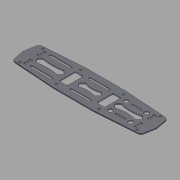
# Autodesk Inventor part: Top Plate
Saved by Autodesk Inventor 2011 SP2 (Build 150309200, 309)
## iProperties
Created: 2015-02-19
Part Number: Top Plate
Document SubType Name: Modeling
Designer: Greg Pavlik
Density: 1 g/cm^3
Author: Greg Pavlik
Autodesk Inventor part; units mm, degrees
ref_plane "YZ Plane" through (0, 0, 0) normal (1, 0, 0) x (0, 1, 0)
ref_plane "XZ Plane" through (0, 0, 0) normal (0, 1, 0) x (-1, 0, 0)
ref_plane "XY Plane" through (0, 0, 0) normal (0, 0, 1) x (1, 0, 0)
sketch "Sketch1" plane through (0, 0, 0) normal (0, 0, 1) x (1, 0, 0)
  line L0 (-92, 0) -> (92, 0) construction
  line L1 (0, 23) -> (0, -23) construction
  line L2 (26.8254, 23) -> (-26.8254, 23)
  line L3 (-27.1742, 22.9878) -> (-84.8084, 18.9576)
  line L4 (-89.3836, 14.8381) -> (-91.8469, 0.8682)
  line L5 (27.1742, 22.9878) -> (84.8084, 18.9576)
  line L6 (89.3836, 14.8381) -> (91.8469, 0.8682)
  line L7 (26.8254, -23) -> (-26.8254, -23)
  line L8 (-27.1742, -22.9878) -> (-84.8084, -18.9576)
  line L9 (-89.3836, -14.8381) -> (-91.8469, -0.8682)
  line L10 (89.3836, -14.8381) -> (91.8469, -0.8682)
  line L11 (27.1742, -22.9878) -> (84.8084, -18.9576)
  arc A0 (-84.8084, 18.9576) -> (-89.3836, 14.8381) centre (-84.4596, 13.9698) ccw
  arc A1 (-26.8254, 23) -> (-27.1742, 22.9878) centre (-26.8254, 18) ccw
  arc A2 (-91.8469, 0.8682) -> (-91.8469, -0.8682) centre (-86.9229, 0) ccw
  arc A3 (-89.3836, -14.8381) -> (-84.8084, -18.9576) centre (-84.4596, -13.9698) ccw
  arc A4 (-27.1742, -22.9878) -> (-26.8254, -23) centre (-26.8254, -18) ccw
  arc A5 (26.8254, -23) -> (27.1742, -22.9878) centre (26.8254, -18) ccw
  arc A6 (84.8084, -18.9576) -> (89.3836, -14.8381) centre (84.4596, -13.9698) ccw
  arc A7 (91.8469, -0.8682) -> (91.8469, 0.8682) centre (86.9229, 0) ccw
  arc A8 (89.3836, 14.8381) -> (84.8084, 18.9576) centre (84.4596, 13.9698) ccw
  arc A9 (27.1742, 22.9878) -> (26.8254, 23) centre (26.8254, 18) ccw
  point P0 (0, 0)
  point P1 (27, 23)
  point P2 (-27, 23)
  point P3 (-88.7053, 18.6851)
  point P4 (88.7053, 18.6851)
  point P5 (27, -23)
  point P6 (-27, -23)
  point P7 (-88.7053, -18.6851)
  point P8 (88.7053, -18.6851)
  dimension "d0" = 184
  dimension "d1" = 54
  dimension "d2" = 46
  dimension "d3" = 160
  dimension "d4" = 8
  dimension "d5" = 5
  constraints: 24 end point, 20 point on circle, 20 point on line, 20 tangent, 10 centre point, 9 equal radius, 7 symmetric about line, 4 midpoint, 2 perpendicular, 1 horizontal
  measures "d0" distance of L0.end L0.start
  measures "d1" distance of point (27, -23) point (-27, -23)
  measures "d2" distance between parallel lines of L2 L7
  measures "d3" angle of L10 L6
  measures "d4" angle of L8 L3
  measures "d5" radius of A0
extrude "Extrusion1" add sketch "Sketch1" along normal mid plane 1.5
sketch "Sketch2" plane through (0, 0, 0.75) normal (0, 0, 1) x (1, 0, 0)
  arc A0 (-91.8469, 0.8682) -> (-91.8469, -0.8682) centre (-86.9229, 0) ccw construction
  line L0 (26.8254, -23) -> (-26.8254, -23) construction
  arc A1 (91.8469, -0.8682) -> (91.8469, 0.8682) centre (86.9229, 0) ccw construction
  line L1 (-26.8254, 23) -> (26.8254, 23) construction
  line L2 (-91.9229, 0) -> (91.9229, 0) construction
  line L3 (0, -23) -> (0, 23) construction
  line L4 (-13, 11.5) -> (13, 11.5)
  line L5 (13, 14.5) -> (-13, 14.5)
  arc A2 (-13, 14.5) -> (-13, 11.5) centre (-13, 13) ccw
  arc A3 (13, 11.5) -> (13, 14.5) centre (13, 13) ccw
  line L6 (-13, -11.5) -> (13, -11.5)
  line L7 (13, -14.5) -> (-13, -14.5)
  arc A4 (-13, -11.5) -> (-13, -14.5) centre (-13, -13) ccw
  arc A5 (13, -14.5) -> (13, -11.5) centre (13, -13) ccw
  line L8 (-30.5, -11.25) -> (-21.5, -11.25)
  line L9 (-20.5, -10.25) -> (-20.5, 10.25)
  line L10 (-21.5, 11.25) -> (-30.5, 11.25)
  line L11 (-31.5, 10.25) -> (-31.5, -10.25)
  arc A6 (-31.5, -10.25) -> (-30.5, -11.25) centre (-30.5, -10.25) ccw
  arc A7 (-21.5, -11.25) -> (-20.5, -10.25) centre (-21.5, -10.25) ccw
  arc A8 (-20.5, 10.25) -> (-21.5, 11.25) centre (-21.5, 10.25) ccw
  arc A9 (-30.5, 11.25) -> (-31.5, 10.25) centre (-30.5, 10.25) ccw
  line L12 (30.5, -11.25) -> (21.5, -11.25)
  line L13 (20.5, -10.25) -> (20.5, 10.25)
  line L14 (21.5, 11.25) -> (30.5, 11.25)
  line L15 (31.5, 10.25) -> (31.5, -10.25)
  arc A10 (30.5, -11.25) -> (31.5, -10.25) centre (30.5, -10.25) ccw
  arc A11 (20.5, -10.25) -> (21.5, -11.25) centre (21.5, -10.25) ccw
  arc A12 (21.5, 11.25) -> (20.5, 10.25) centre (21.5, 10.25) ccw
  arc A13 (31.5, 10.25) -> (30.5, 11.25) centre (30.5, 10.25) ccw
  line L16 (-77, 4.5) -> (-75, 4.5)
  line L17 (-75, 6.5) -> (-75, 12.5)
  line L18 (-75, 14.5) -> (-77, 14.5)
  line L19 (-77, 12.5) -> (-77, 6.5)
  arc A14 (-75, 4.5) -> (-75, 6.5) centre (-75, 5.5) ccw
  arc A15 (-75, 12.5) -> (-75, 14.5) centre (-75, 13.5) ccw
  arc A16 (-77, 14.5) -> (-77, 12.5) centre (-77, 13.5) ccw
  arc A17 (-77, 6.5) -> (-77, 4.5) centre (-77, 5.5) ccw
  line L20 (-77, -4.5) -> (-75, -4.5)
  line L21 (-75, -6.5) -> (-75, -12.5)
  line L22 (-75, -14.5) -> (-77, -14.5)
  line L23 (-77, -12.5) -> (-77, -6.5)
  arc A18 (-75, -6.5) -> (-75, -4.5) centre (-75, -5.5) ccw
  arc A19 (-75, -14.5) -> (-75, -12.5) centre (-75, -13.5) ccw
  arc A20 (-77, -12.5) -> (-77, -14.5) centre (-77, -13.5) ccw
  arc A21 (-77, -4.5) -> (-77, -6.5) centre (-77, -5.5) ccw
  line L24 (77, 4.5) -> (75, 4.5)
  line L25 (75, 6.5) -> (75, 12.5)
  line L26 (75, 14.5) -> (77, 14.5)
  line L27 (77, 12.5) -> (77, 6.5)
  arc A22 (75, 6.5) -> (75, 4.5) centre (75, 5.5) ccw
  arc A23 (75, 14.5) -> (75, 12.5) centre (75, 13.5) ccw
  arc A24 (77, 12.5) -> (77, 14.5) centre (77, 13.5) ccw
  arc A25 (77, 4.5) -> (77, 6.5) centre (77, 5.5) ccw
  arc A26 (75, -4.5) -> (75, -6.5) centre (75, -5.5) ccw
  line L28 (75, -6.5) -> (75, -12.5)
  line L29 (77, -4.5) -> (75, -4.5)
  line L30 (77, -12.5) -> (77, -6.5)
  arc A27 (77, -6.5) -> (77, -4.5) centre (77, -5.5) ccw
  line L31 (75, -14.5) -> (77, -14.5)
  arc A28 (77, -14.5) -> (77, -12.5) centre (77, -13.5) ccw
  arc A29 (75, -12.5) -> (75, -14.5) centre (75, -13.5) ccw
  line L32 (47, 10) -> (59.5, 10)
  line L33 (59.5, 12) -> (47, 12)
  arc A30 (47, 12) -> (47, 10) centre (47, 11) ccw
  arc A31 (59.5, 10) -> (59.5, 12) centre (59.5, 11) ccw
  line L34 (47, -10) -> (59.5, -10)
  line L35 (59.5, -12) -> (47, -12)
  arc A32 (47, -10) -> (47, -12) centre (47, -11) ccw
  arc A33 (59.5, -12) -> (59.5, -10) centre (59.5, -11) ccw
  line L36 (-68, -14.5) -> (-40, -14.5)
  line L37 (-40, -11.5) -> (-68, -11.5)
  arc A34 (-68, -11.5) -> (-68, -14.5) centre (-68, -13) ccw
  arc A35 (-40, -14.5) -> (-40, -11.5) centre (-40, -13) ccw
  line L38 (-68, 14.5) -> (-40, 14.5)
  line L39 (-40, 11.5) -> (-68, 11.5)
  arc A36 (-68, 14.5) -> (-68, 11.5) centre (-68, 13) ccw
  arc A37 (-40, 11.5) -> (-40, 14.5) centre (-40, 13) ccw
  point P0 (0, 0)
  dimension "d8" = 1.5
  dimension "d9" = 26
  dimension "d10" = 26
  dimension "d11" = 1
  dimension "d12" = 22.5
  dimension "d13" = 11
  dimension "d14" = 41
  dimension "d15" = 9
  dimension "d16" = 10
  dimension "d17" = 2
  dimension "d18" = 1
  dimension "d19" = 75
  dimension "d20" = 22
  dimension "d21" = 1
  dimension "d22" = 12.5
  dimension "d23" = 47
  dimension "d24" = 28
  dimension "d25" = 1.5
  dimension "d26" = 40
  dimension "d27" = 26
  constraints: 76 end point, 74 point on circle, 66 symmetric about line, 36 centre point, 24 tangent, 16 point on line, 7 parallel, 6 equal radius, 5 horizontal, 2 midpoint, 2 perpendicular, 24 other
  measures "d8" radius of A3
  measures "d9" distance of A2.centre A4.centre
  measures "d10" distance of A3.centre A2.centre
  measures "d11" radius of A6
  measures "d12" distance between parallel lines of L10 L8
  measures "d13" distance between parallel lines of L9 L11
  measures "d14" distance between parallel lines of L9 L13
  measures "d15" distance between parallel lines of L16 L20
  measures "d16" distance between parallel lines of L22 L20
  measures "d17" distance between parallel lines of L21 L23
  measures "d18" radius of A19
  measures "d19" distance between parallel lines of L3 L21
  measures "d20" distance of A30.centre A32.centre
  measures "d21" radius of A31
  measures "d22" distance of A31.centre A30.centre
  measures "d23" distance from line of L3 A30.centre
  measures "d24" distance of A35.centre A34.centre
  measures "d25" radius of A34
  measures "d26" distance from line of L3 A35.centre
  measures "d27" distance of A36.centre A34.centre
extrude "Extrusion2" cut sketch "Sketch2" against normal through all
sketch "Sketch3" plane through (0, 0, 0.75) normal (0, 0, 1) x (1, 0, 0)
  arc A0 (-91.8469, 0.8682) -> (-91.8469, -0.8682) centre (-86.9229, 0) ccw construction
  arc A1 (91.8469, -0.8682) -> (91.8469, 0.8682) centre (86.9229, 0) ccw construction
  line L0 (-26.8254, 23) -> (26.8254, 23) construction
  line L1 (-86.9229, 0) -> (86.9229, 0) construction
  line L2 (0, -31.5) -> (0, 31.5) construction
  line L3 (53.25, -53.5) -> (53.25, 53.5) construction
  line L4 (-55, -70.6875) -> (-55, 70.6875) construction
  arc A2 (39.3923, 4.4188) -> (67.1077, 4.4188) centre (53.25, 53.5) ccw
  arc A3 (67.1077, -4.4188) -> (39.3923, -4.4188) centre (53.25, -53.5) ccw
  line L5 (68.0865, -4.1635) -> (71.5429, -0.7071)
  line L6 (38.4135, -4.1635) -> (34.9571, -0.7071)
  line L7 (68.0865, 4.1635) -> (71.5429, 0.7071)
  line L8 (38.4135, 4.1635) -> (34.9571, 0.7071)
  arc A4 (10.2822, -4.384) -> (-10.2822, -4.384) centre (0, -31.5) ccw
  arc A5 (-10.2822, 4.384) -> (10.2822, 4.384) centre (0, 31.5) ccw
  line L9 (11.3439, -4.1561) -> (14.7929, -0.7071)
  line L10 (14.7929, 0.7071) -> (11.3439, 4.1561)
  line L11 (-11.3439, -4.1561) -> (-14.7929, -0.7071)
  line L12 (-14.7929, 0.7071) -> (-11.3439, 4.1561)
  arc A6 (-41.2432, -4.6042) -> (-68.7568, -4.6042) centre (-55, -70.6875) ccw
  arc A7 (-68.7568, 4.6042) -> (-41.2432, 4.6042) centre (-55, 70.6875) ccw
  line L13 (-69.6677, -4.3323) -> (-73.2929, -0.7071)
  line L14 (-73.2929, 0.7071) -> (-69.6677, 4.3323)
  line L15 (-40.3323, -4.3323) -> (-36.7071, -0.7071)
  line L16 (-36.7071, 0.7071) -> (-40.3323, 4.3323)
  arc A8 (39.3923, 4.4188) -> (38.4135, 4.1635) centre (39.1206, 3.4564) ccw
  arc A9 (34.9571, 0.7071) -> (34.9571, -0.7071) centre (35.6642, 0) ccw
  arc A10 (38.4135, -4.1635) -> (39.3923, -4.4188) centre (39.1206, -3.4564) ccw
  arc A11 (67.1077, -4.4188) -> (68.0865, -4.1635) centre (67.3794, -3.4564) ccw
  arc A12 (71.5429, -0.7071) -> (71.5429, 0.7071) centre (70.8358, 0) ccw
  arc A13 (68.0865, 4.1635) -> (67.1077, 4.4188) centre (67.3794, 3.4564) ccw
  arc A14 (14.7929, -0.7071) -> (14.7929, 0.7071) centre (14.0858, 0) ccw
  arc A15 (11.3439, 4.1561) -> (10.2822, 4.384) centre (10.6368, 3.449) ccw
  arc A16 (10.2822, -4.384) -> (11.3439, -4.1561) centre (10.6368, -3.449) ccw
  arc A17 (-11.3439, -4.1561) -> (-10.2822, -4.384) centre (-10.6368, -3.449) ccw
  arc A18 (-14.7929, 0.7071) -> (-14.7929, -0.7071) centre (-14.0858, 0) ccw
  arc A19 (-10.2822, 4.384) -> (-11.3439, 4.1561) centre (-10.6368, 3.449) ccw
  arc A20 (-36.7071, -0.7071) -> (-36.7071, 0.7071) centre (-37.4142, 0) ccw
  arc A21 (-41.2432, -4.6042) -> (-40.3323, -4.3323) centre (-41.0394, -3.6252) ccw
  arc A22 (-40.3323, 4.3323) -> (-41.2432, 4.6042) centre (-41.0394, 3.6252) ccw
  arc A23 (-68.7568, 4.6042) -> (-69.6677, 4.3323) centre (-68.9606, 3.6252) ccw
  arc A24 (-69.6677, -4.3323) -> (-68.7568, -4.6042) centre (-68.9606, -3.6252) ccw
  arc A25 (-73.2929, 0.7071) -> (-73.2929, -0.7071) centre (-72.5858, 0) ccw
  point P0 (0, 0)
  point P1 (72.25, 0)
  point P2 (34.25, 0)
  point P3 (67.6692, 4.5808)
  point P4 (38.8308, 4.5808)
  point P5 (38.8308, -4.5808)
  point P6 (67.6692, -4.5808)
  point P7 (15.5, 0)
  point P8 (-15.5, 0)
  point P9 (-10.8812, 4.6188)
  point P10 (10.8812, 4.6188)
  point P11 (10.8812, -4.6188)
  point P12 (-10.8812, -4.6188)
  point P13 (-74, 0)
  point P14 (-36, 0)
  point P15 (-69.2839, -4.7161)
  point P16 (-40.7161, -4.7161)
  point P17 (-69.2839, 4.7161)
  point P18 (-40.7161, 4.7161)
  dimension "d30" = 53.25
  dimension "d31" = 55
  dimension "d32" = 107
  dimension "d33" = 51
  dimension "d34" = 63
  dimension "d35" = 29
  dimension "d36" = 67.5
  dimension "d37" = 141.375
  dimension "d38" = 38
  dimension "d39" = 31
  dimension "d40" = 38
  dimension "d41" = 1
  constraints: 60 point on circle, 36 tangent, 32 end point, 28 point on line, 24 centre point, 17 equal radius, 6 coincident, 5 perpendicular, 5 symmetric about line, 3 parallel, 2 midpoint, 15 other
  measures "d30" distance between parallel lines of L3 L2
  measures "d31" distance between parallel lines of L4 L2
  measures "d32" distance of L3.end L3.start
  measures "d33" radius of A2
  measures "d34" distance of L2.end L2.start
  measures "d35" radius of A5
  measures "d36" radius of A7
  measures "d37" distance of L4.end L4.start
  measures "d38" distance of point (-36, 0) point (-74, 0)
  measures "d39" distance of point (15.5, 0) point (-15.5, 0)
  measures "d40" distance of point (72.25, 0) point (34.25, 0)
  measures "d41" radius of A8
extrude "Extrusion3" cut sketch "Sketch3" against normal through all
sketch "Sketch4" plane through (0, 0, 0.75) normal (0, 0, 1) x (1, 0, 0)
  line L0 (26.8254, -23) -> (-26.8254, -23) construction
  line L1 (-26.8254, 23) -> (26.8254, 23) construction
  line L2 (0, -23) -> (0, 23) construction
  line L3 (39.25, -11) -> (67.25, -11)
  line L4 (67.25, -11) -> (67.25, 11)
  line L5 (67.25, 11) -> (39.25, 11)
  line L6 (39.25, 11) -> (39.25, -11)
  line L7 (0, 0) -> (26.8254, 0) construction
  dimension "d44" = 22
  dimension "d45" = 28
  dimension "d46" = 39.25
  constraints: 13 end point, 3 coincident, 2 midpoint, 2 parallel, 2 perpendicular, 1 horizontal, 1 other
  measures "d44" distance between parallel lines of L5 L3
  measures "d45" distance between parallel lines of L4 L6
  measures "d46" distance between parallel lines of L2 L6
hole "Hole1" at (39.25, -11, 0.75) at (39.25, 11, 0.75) at (67.25, 11, 0.75) at (67.25, -11, 0.75) direction (0, 0, -1) diameter 6 end through all
sketch "Sketch5" plane through (0, 0, 0.75) normal (0, 0, 1) x (1, 0, 0)
  line L0 (0, 0) -> (0, 24.6505)
  line L1 (0, 0) -> (42.2762, 0)
  point P0 (81, 16)
  point P1 (81, -16)
  point P2 (29.5, 17)
  point P3 (29.5, -17)
  point P4 (-29.5, 17)
  point P5 (-29.5, -17)
  point P6 (-81, 16)
  point P7 (-81, -16)
  dimension "d54" = 32
  dimension "d55" = 51.5
  dimension "d56" = 34
  dimension "d57" = 59
  constraints: 6 symmetric about line, 4 end point, 1 perpendicular, 1 vertical
  measures "d54" distance of point (81, 16) point (81, -16)
  measures "d55" horizontal distance of point (81, -16) point (29.5, -17)
  measures "d56" distance of point (29.5, 17) point (29.5, -17)
  measures "d57" distance of point (-29.5, -17) point (29.5, -17)
hole "Hole2" at (81, 16, 0.75) at (81, -16, 0.75) at (29.5, 17, 0.75) at (29.5, -17, 0.75) at (-29.5, 17, 0.75) at (-29.5, -17, 0.75) at (-81, 16, 0.75) at (-81, -16, 0.75) direction (0, 0, -1) diameter 3 end through all
chamfer "Chamfer1" distance 0.15 angle 45 72 edges at (53.25, -2.5, 0.75) (38.8683, -4.424, 0.75) (36.6853, -2.4353, 0.75) (34.6642, 0, 0.75) (36.6853, 2.4353, 0.75) (38.8683, 4.424, 0.75) (53.25, 2.5, 0.75) (67.6317, 4.424, 0.75) (69.8147, 2.4353, 0.75) (71.8358, 0, 0.75) (69.8147, -2.4353, 0.75) (67.6317, -4.424, 0.75) (53.25, -2.5, -0.75) (67.6317, -4.424, -0.75) (69.8147, -2.4353, -0.75) (71.8358, 0, -0.75) (69.8147, 2.4353, -0.75) (67.6317, 4.424, -0.75) (53.25, 2.5, -0.75) (38.8683, 4.424, -0.75) (36.6853, 2.4353, -0.75) (34.6642, 0, -0.75) (36.6853, -2.4353, -0.75) (38.8683, -4.424, -0.75) (0, -2.5, -0.75) (10.8467, -4.4267, -0.75) (13.0684, -2.4316, -0.75) (15.0858, 0, -0.75) (13.0684, 2.4316, -0.75) (10.8467, 4.4267, -0.75) (0, 2.5, -0.75) (-10.8467, 4.4267, -0.75) (-13.0684, 2.4316, -0.75) (-15.0858, 0, -0.75) (-13.0684, -2.4316, -0.75) (-10.8467, -4.4267, -0.75) (0, -2.5, 0.75) (-10.8467, -4.4267, 0.75) (-13.0684, -2.4316, 0.75) (-15.0858, 0, 0.75) (-13.0684, 2.4316, 0.75) (-10.8467, 4.4267, 0.75) (0, 2.5, 0.75) (10.8467, 4.4267, 0.75) (13.0684, 2.4316, 0.75) (15.0858, 0, 0.75) (13.0684, -2.4316, 0.75) (10.8467, -4.4267, 0.75) (-55, -3.1875, -0.75) (-40.7534, -4.5834, -0.75) (-38.5197, -2.5197, -0.75) (-36.4142, 0, -0.75) (-38.5197, 2.5197, -0.75) (-40.7534, 4.5834, -0.75) (-55, 3.1875, -0.75) (-69.2466, 4.5834, -0.75) (-71.4803, 2.5197, -0.75) (-73.5858, 0, -0.75) (-71.4803, -2.5197, -0.75) (-69.2466, -4.5834, -0.75) (-55, -3.1875, 0.75) (-69.2466, -4.5834, 0.75) (-71.4803, -2.5197, 0.75) (-73.5858, 0, 0.75) (-71.4803, 2.5197, 0.75) (-69.2466, 4.5834, 0.75) (-55, 3.1875, 0.75) (-40.7534, 4.5834, 0.75) (-38.5197, 2.5197, 0.75) (-36.4142, 0, 0.75) (-38.5197, -2.5197, 0.75) (-40.7534, -4.5834, 0.75)
chamfer "Chamfer2" distance 0.15 angle 45 80 edges at (-54, 11.5, -0.75) (-38.5, 13, -0.75) (-54, 14.5, -0.75) (-69.5, 13, -0.75) (-54, 11.5, 0.75) (-69.5, 13, 0.75) (-54, 14.5, 0.75) (-38.5, 13, 0.75) (-54, -14.5, 0.75) (-69.5, -13, 0.75) (-54, -11.5, 0.75) (-38.5, -13, 0.75) (-54, -14.5, -0.75) (-38.5, -13, -0.75) (-54, -11.5, -0.75) (-69.5, -13, -0.75) (-26, -11.25, 0.75) (-31.2071, -10.9571, 0.75) (-31.5, 0, 0.75) (-31.2071, 10.9571, 0.75) (-26, 11.25, 0.75) (-20.7929, 10.9571, 0.75) (-20.5, 0, 0.75) (-20.7929, -10.9571, 0.75) (-26, -11.25, -0.75) (-20.7929, -10.9571, -0.75) (-20.5, 0, -0.75) (-20.7929, 10.9571, -0.75) (-26, 11.25, -0.75) (-31.2071, 10.9571, -0.75) (-31.5, 0, -0.75) (-31.2071, -10.9571, -0.75) (-14.5, -13, 0.75) (0, -11.5, 0.75) (14.5, -13, 0.75) (0, -14.5, 0.75) (0, -14.5, -0.75) (14.5, -13, -0.75) (0, -11.5, -0.75) (-14.5, -13, -0.75) (0, 11.5, 0.75) (-14.5, 13, 0.75) (0, 14.5, 0.75) (14.5, 13, 0.75) (0, 11.5, -0.75) (14.5, 13, -0.75) (0, 14.5, -0.75) (-14.5, 13, -0.75) (20.5, 0, -0.75) (20.7929, -10.9571, -0.75) (26, -11.25, -0.75) (31.2071, -10.9571, -0.75) (31.5, 0, -0.75) (31.2071, 10.9571, -0.75) (26, 11.25, -0.75) (20.7929, 10.9571, -0.75) (20.5, 0, 0.75) (20.7929, 10.9571, 0.75) (26, 11.25, 0.75) (31.2071, 10.9571, 0.75) (31.5, 0, 0.75) (31.2071, -10.9571, 0.75) (26, -11.25, 0.75) (20.7929, -10.9571, 0.75) (53.25, -12, 0.75) (46, -11, 0.75) (53.25, -10, 0.75) (60.5, -11, 0.75) (53.25, -10, -0.75) (46, -11, -0.75) (53.25, -12, -0.75) (60.5, -11, -0.75) (53.25, 12, 0.75) (60.5, 11, 0.75) (53.25, 10, 0.75) (46, 11, 0.75) (53.25, 12, -0.75) (46, 11, -0.75) (53.25, 10, -0.75) (60.5, 11, -0.75)
chamfer "Chamfer3" distance 0.15 angle 45 64 edges at (76, -14.5, 0.75) (74, -13.5, 0.75) (78, -13.5, 0.75) (76, -14.5, -0.75) (78, -13.5, -0.75) (74, -13.5, -0.75) (75, -9.5, -0.75) (75, -9.5, 0.75) (74, -5.5, 0.75) (76, -4.5, 0.75) (78, -5.5, 0.75) (74, -5.5, -0.75) (76, -4.5, -0.75) (78, -5.5, -0.75) (77, -9.5, 0.75) (77, -9.5, -0.75) (77, 9.5, 0.75) (75, 9.5, 0.75) (75, 9.5, -0.75) (77, 9.5, -0.75) (78, 5.5, 0.75) (76, 4.5, 0.75) (74, 5.5, 0.75) (78, 5.5, -0.75) (76, 4.5, -0.75) (74, 5.5, -0.75) (76, 14.5, 0.75) (78, 13.5, 0.75) (74, 13.5, 0.75) (76, 14.5, -0.75) (74, 13.5, -0.75) (78, 13.5, -0.75) (-76, 14.5, -0.75) (-78, 13.5, -0.75) (-74, 13.5, -0.75) (-78, 13.5, 0.75) (-76, 14.5, 0.75) (-74, 13.5, 0.75) (-77, 9.5, 0.75) (-77, 9.5, -0.75) (-75, 9.5, 0.75) (-75, 9.5, -0.75) (-78, 5.5, -0.75) (-76, 4.5, -0.75) (-74, 5.5, -0.75) (-76, 4.5, 0.75) (-78, 5.5, 0.75) (-74, 5.5, 0.75) (-76, -4.5, 0.75) (-74, -5.5, 0.75) (-78, -5.5, 0.75) (-76, -4.5, -0.75) (-78, -5.5, -0.75) (-74, -5.5, -0.75) (-77, -9.5, -0.75) (-77, -9.5, 0.75) (-76, -14.5, 0.75) (-78, -13.5, 0.75) (-74, -13.5, 0.75) (-76, -14.5, -0.75) (-74, -13.5, -0.75) (-78, -13.5, -0.75) (-75, -9.5, 0.75) (-75, -9.5, -0.75)
chamfer "Chamfer4" distance 0.15 angle 45 16 edges at (-81, -14.5, 0.75) (-29.5, -15.5, 0.75) (29.5, -15.5, 0.75) (81, -14.5, 0.75) (-81, 17.5, 0.75) (-29.5, 18.5, 0.75) (29.5, 18.5, 0.75) (81, 17.5, 0.75) (-81, -14.5, -0.75) (-29.5, -15.5, -0.75) (29.5, -15.5, -0.75) (81, -14.5, -0.75) (-81, 17.5, -0.75) (-29.5, 18.5, -0.75) (29.5, 18.5, -0.75) (81, 17.5, -0.75)
chamfer "Chamfer5" distance 0.15 angle 45 8 edges at (39.25, -8, 0.75) (67.25, -8, 0.75) (39.25, 14, 0.75) (67.25, 14, 0.75) (39.25, -8, -0.75) (67.25, -8, -0.75) (39.25, 14, -0.75) (67.25, 14, -0.75)
chamfer "Chamfer6" distance 0.15 angle 45 40 edges at (90.6153, 7.8532, 0.75) (91.9229, 0, 0.75) (90.6153, -7.8532, 0.75) (87.8053, -17.6855, 0.75) (55.9913, -20.9727, 0.75) (26.9999, -22.997, 0.75) (0, -23, 0.75) (-26.9999, -22.997, 0.75) (-55.9913, -20.9727, 0.75) (-87.8053, -17.6855, 0.75) (-90.6153, -7.8532, 0.75) (-91.9229, 0, 0.75) (-90.6153, 7.8532, 0.75) (-87.8053, 17.6855, 0.75) (-55.9913, 20.9727, 0.75) (-26.9999, 22.997, 0.75) (0, 23, 0.75) (26.9999, 22.997, 0.75) (55.9913, 20.9727, 0.75) (87.8053, 17.6855, 0.75) (90.6153, 7.8532, -0.75) (87.8053, 17.6855, -0.75) (55.9913, 20.9727, -0.75) (26.9999, 22.997, -0.75) (0, 23, -0.75) (-26.9999, 22.997, -0.75) (-55.9913, 20.9727, -0.75) (-87.8053, 17.6855, -0.75) (-90.6153, 7.8532, -0.75) (-91.9229, 0, -0.75) (-90.6153, -7.8532, -0.75) (-87.8053, -17.6855, -0.75) (-55.9913, -20.9727, -0.75) (-26.9999, -22.997, -0.75) (0, -23, -0.75) (26.9999, -22.997, -0.75) (55.9913, -20.9727, -0.75) (87.8053, -17.6855, -0.75) (90.6153, -7.8532, -0.75) (91.9229, 0, -0.75)
body "Solid1"
